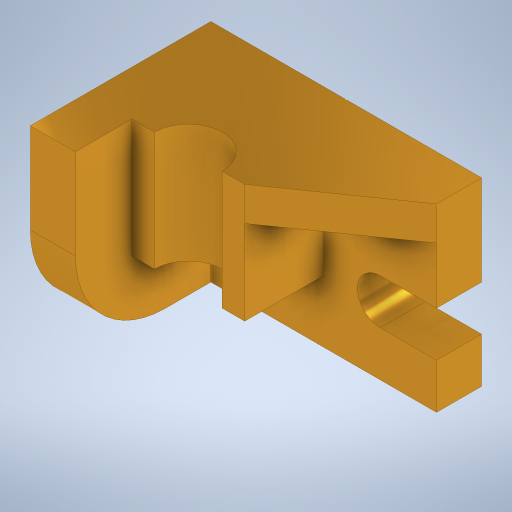
# Autodesk Inventor part: Exercise 1
Saved by Autodesk Inventor 2023 (Build 270158000, 158)
## iProperties
Created: 2023-02-02
Part Number: Exercise 1
Material: Glass
Document SubType Name: Modeling
Designer: General
Density: 2.18 g/cm^3
Appearance: Metal 1800F Hot
Author: General
Autodesk Inventor part; units mm, degrees
ref_plane "YZ Plane" through (0, 0, 0) normal (1, 0, 0) x (0, 1, 0)
ref_plane "XZ Plane" through (0, 0, 0) normal (0, 1, 0) x (-1, 0, 0)
ref_plane "XY Plane" through (0, 0, 0) normal (0, 0, 1) x (1, 0, 0)
sketch "Sketch1" plane through (0, 0, 0) normal (0, 0, 1) x (1, 0, 0)
  line L0 (48, 32) -> (-48, 32)
  line L1 (-48, 32) -> (-48, -32)
  line L2 (-48, -32) -> (48, -32)
  line L3 (48, -32) -> (48, 32)
  line L4 (48, 32) -> (-48, -32) construction
  line L5 (-48, 32) -> (48, -32) construction
  point P0 (0, 0)
  dimension "d0" = 96
  dimension "d1" = 64
  constraints: 12 end point, 2 midpoint, 2 parallel, 1 horizontal, 1 perpendicular
  measures "d0" distance of L2.end L1.end
  measures "d1" distance of L1.end L0.end
extrude "Extrusion1" add sketch "Sketch1" along normal blind 16
sketch "Sketch2" plane through (0, 0, 16) normal (0, 0, 1) x (1, 0, 0)
  line L0 (-48, 32) -> (-48, -32) projected
  line L1 (-48, 32) -> (-32, 32)
  line L2 (-32, 32) -> (-32, -32)
  line L3 (-32, -32) -> (-48, -32)
  line L4 (-48, -32) -> (-48, 32)
  line L5 (-48, -32) -> (48, -32) projected
  point P0 (0, 0)
  dimension "d4" = 16
  constraints: 8 end point, 2 parallel, 1 collinear, 1 horizontal, 1 perpendicular
  measures "d4" distance of L2.end L3.end
extrude "Extrusion2" add sketch "Sketch2" along normal blind 48
fillet "Fillet1" radius 32 1 edges at (-40, -32, 64)
sketch "Sketch3" plane through (-48, 32, 0) normal (0, 1, 0) x (1, 0, 0)
  point P0 (48, 0)
sketch "Sketch4" plane through (-48, 32, 0) normal (0, 1, 0) x (1, 0, 0)
  point P0 (48, 0)
sketch "Sketch5" plane through (-48, 32, 0) normal (0, 1, 0) x (1, 0, 0)
  line L0 (16, -16) -> (96, -16) projected
  line L1 (16, -16) -> (56, -16)
  line L2 (56, -16) -> (56, -44)
  line L3 (16, -44) -> (16, -16)
  arc A0 (48, -44) -> (24, -44) centre (36, -44) ccw
  line L4 (56, -44) -> (48, -44)
  line L5 (24, -44) -> (16, -44)
  point P0 (48, 0)
  dimension "d8" = 40
  dimension "d9" = 28
  dimension "d10" = 24
  constraints: 10 end point, 3 parallel, 2 point on circle, 1 centre point, 1 horizontal, 1 perpendicular
  measures "d8" distance of L2.end L3.start
  measures "d9" distance of L1.end L2.end
  measures "d10" diameter of A0
extrude "Extrusion3" add sketch "Sketch5" against normal blind 42
sketch "Sketch6" plane through (-48, 32, 0) normal (0, 1, 0) x (1, 0, 0)
  line L0 (48, -44) -> (56, -44) projected
  line L1 (96, -16) -> (56, -16) projected
  line L2 (56, -44) -> (96, -16)
  line L3 (96, -16) -> (56, -16)
  line L4 (56, -16) -> (56, -44) projected
  line L5 (56, -16) -> (56, -44)
  point P0 (48, 0)
  constraints: 6 end point, 2 collinear
extrude "Extrusion4" add sketch "Sketch6" against normal blind 12
sketch "Sketch7" plane through (0, 0, 16) normal (0, 0, 1) x (1, 0, 0)
  line L0 (48, -32) -> (48, 32) projected
  line L1 (48, -16) -> (28, -16)
  arc A0 (28, 0) -> (28, -16) centre (28, -8) ccw
  line L2 (28, 0) -> (48, 0)
  point P0 (0, 0)
  dimension "d15" = 20
  dimension "d16" = 16
  dimension "d17" = 16
  constraints: 4 end point, 2 point on circle, 2 tangent, 1 centre point, 1 horizontal, 1 midpoint, 1 parallel, 1 point on line
  measures "d15" distance of L1.start L1.end
  measures "d16" distance of L2.start L1.end
  measures "d17" distance of L1.start L0.start
extrude "Extrusion5" cut sketch "Sketch7" against normal blind 16
body "Solid1"
